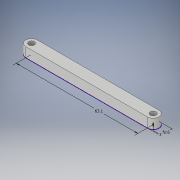
# Autodesk Inventor part: test5
Saved by Autodesk Inventor 2019 (Build 230136000, 136)
## iProperties
Created: 2021-02-06
Part Number: test5
Material: 一般
Document SubType Name: Modeling
Designer: wasd5
Density: 1 g/cm^3
Appearance: 預設
Author: wasd5
Autodesk Inventor part; units mm, degrees
ref_plane "YZ Plane" through (0, 0, 0) normal (1, 0, 0) x (0, 1, 0)
ref_plane "XZ Plane" through (0, 0, 0) normal (0, 1, 0) x (-1, 0, 0)
ref_plane "XY Plane" through (0, 0, 0) normal (0, 0, 1) x (1, 0, 0)
sketch "草圖3" plane through (0, 0, 0) normal (0, 1, 0) x (-1, 0, 0)
  line L0 (-66.1, 0) -> (3, 0) construction
  line L1 (-63.1, 3) -> (0, 3)
  line L2 (0, -3) -> (-63.1, -3)
  arc A0 (-63.1, 3) -> (-63.1, -3) centre (-63.1, 0) ccw
  arc A1 (0, -3) -> (0, 3) centre (0, 0) ccw
  circle A2 centre (-63.1, 0) radius 1.5
  circle A3 centre (0, 0) radius 1.5
  point P0 (-31.55, 0)
  dimension "hole" = 3
  dimension "d14" = 6
  dimension "center_distance" = 63.1
  constraints: 8 end point, 6 point on circle, 4 centre point, 4 tangent, 3 coincident, 2 point on line, 1 equal radius, 1 horizontal, 1 midpoint, 1 parallel
  measures "hole" diameter of A2
  measures "d14" distance between parallel lines of L1 L2
  measures "center_distance" distance of A0.centre point (0, 0)
extrude "擠出3" add sketch "草圖3" along normal blind 5
equation "\"d14\" = 2 * hole"
